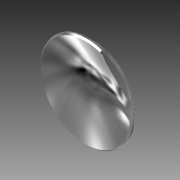
# Autodesk Inventor part: small cap
Saved by Autodesk Inventor 2014 (Build 180170000, 170)
## iProperties
Shininess: 100.0
Length Units: 11272
Angle Units: 11279
Time Units: 11290
Mass Units: 11286
Length Display Precision: 3
Angle Display Precision: 2
Compacted: True
Created: 2001-07-10
Part Number: small cap
Document SubType Name: Modeling
Designer: Autodesk, Inc.
Mass: 0.282551 g
Surface Area: 1.12327 cm^2
Volume: 0.0349692 cm^3
Density: 8.08 g/cm^3
Material: Stainless Steel
Appearance: Black Chrome
Density: 0.0
Volumn: 0.0
Area: 0.0
PropertySet Name: Model Information
Control State: 0
Master: False
Checked Out: False
Author: Autodesk, Inc.
Autodesk Inventor part; units mm, degrees
ref_plane "Work Plane1" through (0, 0, 0) normal (0, 0, 1) x (1, 0, 0)
ref_plane "Work Plane2" through (-6.35, -6.7108, 0.3969) normal (0, 0, 1) x (1, 0, 0)
sketch "Sketch2" plane through (0, 0, 0) normal (0, 0, 1) x (1, 0, 0)
  circle A0 centre (0, -0.3608) radius 3.9687 projected
extrude "Extrusion1" add sketch "Sketch2" along normal up to surface (0.3969 mm away)
chamfer "Chamfer1" distance 0.127 angle 45 1 edges at (-3.9687, -0.3608, 0.3969)
ref_plane "Work Plane3" through (-6.35, -5.917, -0.3969) normal (0, 0, -1) x (0, 1, 0)
sketch "Sketch3" plane through (0, -0.3608, 0) normal (0, 0, -1) x (-1, 0, 0)
  circle A0 centre (0, 0) radius 3.5719 projected
extrude "Extrusion2" add sketch "Sketch3" along normal up to surface (0.3969 mm away)
chamfer "Chamfer2" distance 0.127 angle 45 2 edges at (3.5719, -0.3608, -0.3969) (-3.9687, -0.3608, 0)
body "Solid1"
